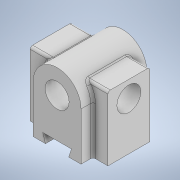
# Autodesk Inventor part: Część9
Saved by Autodesk Inventor 2021 (Build 250183000, 183)
## iProperties
Created: 2023-09-29
Part Number: Część9
Material: Ogólny
Document SubType Name: Modeling
Designer: Jakub
Density: 1 g/cm^3
Appearance: Domyślna
Author: Jakub
Autodesk Inventor part; units mm, degrees
ref_plane "YZ Plane" through (0, 0, 0) normal (1, 0, 0) x (0, 1, 0)
ref_plane "XZ Plane" through (0, 0, 0) normal (0, 1, 0) x (-1, 0, 0)
ref_plane "XY Plane" through (0, 0, 0) normal (0, 0, 1) x (1, 0, 0)
sketch "Szkic1" plane through (0, 0, 0) normal (0, 0, 1) x (1, 0, 0)
  line L0 (0, 0) -> (8, 0)
  line L1 (8, 0) -> (8, 7)
  line L2 (8, 7) -> (32, 7)
  line L3 (32, 7) -> (32, 0)
  line L4 (32, 0) -> (40, 0)
  line L5 (40, 0) -> (40, 60)
  line L6 (40, 60) -> (0, 60)
  line L7 (0, 60) -> (0, 0)
  line L8 (8, 7) -> (10.2744, 0)
  line L9 (8, 7) -> (15.3602, 7) construction
  line L10 (32, 7) -> (29.7256, 0)
  line L11 (32, 7) -> (39.3602, 7) construction
  line L12 (8, 0) -> (10.2744, 0)
  line L13 (29.7256, 0) -> (40, 0)
  dimension "d0" = 8
  dimension "d1" = 7
  dimension "d2" = 24
  dimension "d3" = 8
  dimension "d4" = 60
  dimension "d5" = 90
  dimension "d6" = 72
  dimension "d7" = 108
  constraints: 28 end point, 5 perpendicular, 4 horizontal, 2 equal length, 2 point on line, 1 collinear
  measures "d0" distance of L0.start L0.end
  measures "d1" distance of L0.end L1.end
  measures "d2" distance of L1.end L2.end
  measures "d3" distance of L3.end L4.end
  measures "d4" distance of L4.end L5.end
  measures "d5" angle of L6 L5
  measures "d6" angle of L8 L9
  measures "d7" angle of L10 L11
extrude "Wyciągnięcie proste1" add sketch "Szkic1" along normal blind 55
sketch "Szkic2" plane through (0, 0, 0) normal (-1, 0, 0) x (0, 0, 1)
  line L0 (10, 0) -> (10, 54)
  line L1 (10, 54) -> (45, 54)
  line L2 (45, 54) -> (45, 0)
  line L3 (0, 0) -> (55, 0) projected
  dimension "d10" = 54
  dimension "d11" = 35
  constraints: 6 end point, 2 perpendicular, 1 point on line, 1 vertical
  measures "d10" distance of L0.start L0.end
  measures "d11" distance of L0.end L1.end
sketch "Szkic3" plane through (40, 0, 0) normal (1, 0, 0) x (0, 0, -1)
  line L0 (-45, 0) -> (-45, 54)
  line L1 (0, 60) -> (-55, 60) projected
  line L2 (-10, 54) -> (-45, 54) projected
  line L3 (-45, 54) -> (-10, 54)
  line L4 (-10, 54) -> (-10, 0)
  line L5 (0, 0) -> (-55, 0) projected
  line L6 (-10, 0) -> (-45, 0)
  dimension "d14" = 54
  constraints: 8 end point, 2 perpendicular, 1 collinear, 1 point on line
  measures "d14" distance of L0.start L0.end
extrude "Wyciągnięcie proste3" add sketch "Szkic3" along normal blind 12.5
extrude "Wyciągnięcie proste5" add sketch "Szkic2" along normal blind 12.5
fillet "Zaokrąglenie11" radius 20 1 edges at (40, 60, 27.5)
fillet "Zaokrąglenie12" radius 20 1 edges at (0, 60, 27.5)
fillet "Zaokrąglenie13" radius 2 14 edges at (38.5156, 47.5612, 45) (40, 20, 45) (0, 20, 45) (1.4844, 47.5612, 45) (0, 20, 10) (1.4844, 47.5612, 10) (40, 20, 10) (38.5156, 47.5612, 10) (34.2829, 54, 27.5) (5.7171, 54, 27.5) (-3.3914, 54, 10) (-3.3914, 54, 45) (43.3914, 54, 45) (43.3914, 54, 10)
sketch "Szkic5" plane through (-12.5, 0, 0) normal (-1, 0, 0) x (0, 0, 1)
  line L0 (10, 0) -> (45, 0) projected
  line L1 (27.5, 0) -> (27.5, 40)
  circle A0 centre (27.5, 40) radius 10
  point P0 (0, 0)
  dimension "d34" = 40
  dimension "d35" = 20
  constraints: 2 end point, 1 centre point, 1 coincident, 1 midpoint, 1 vertical
  measures "d34" distance of L1.start L1.end
  measures "d35" diameter of A0
extrude "Wyciągnięcie proste6" cut sketch "Szkic5" against normal blind 65
sketch "Szkic7" plane through (-12.5, 0, 0) normal (-1, 0, 0) x (0, 0, 1)
  line L0 (27.5, 40) -> (18.8964, 27.7127)
  line L1 (27.5, 40) -> (42.5, 40) construction
  line L2 (18.8964, 27.7127) -> (20.5347, 26.5656)
  line L3 (20.5347, 26.5656) -> (23.5184, 30.8268)
  circle A0 centre (27.5, 40) radius 10 projected
  line L4 (18.8964, 27.7127) -> (17.258, 28.8599)
  line L5 (17.258, 28.8599) -> (20.2418, 33.1211)
  point P0 (0, 0)
  dimension "d39" = 15
  dimension "d40" = 125
  dimension "d41" = 2
  dimension "d42" = 2
  constraints: 12 end point, 3 perpendicular, 1 equal length, 1 horizontal, 1 point on line, 2 other
  measures "d39" distance of L0.start L0.end
  measures "d40" angle of L0 L1
  measures "d41" distance of L0.end L2.end
  measures "d42" distance of L0.end L4.end
extrude "Wyciągnięcie proste7" cut sketch "Szkic7" against normal blind 8 contours A0 L3 L2 L0 | L0 L4 L5 A0
sketch "Szkic8" plane through (0, 0, 55) normal (0, 0, 1) x (1, 0, 0)
  circle A0 centre (20, 40) radius 10
  point P0 (0, 0)
  dimension "d45" = 20
  constraints: 1 centre point
  measures "d45" diameter of A0
extrude "Wyciągnięcie proste8" cut sketch "Szkic8" against normal blind 65
